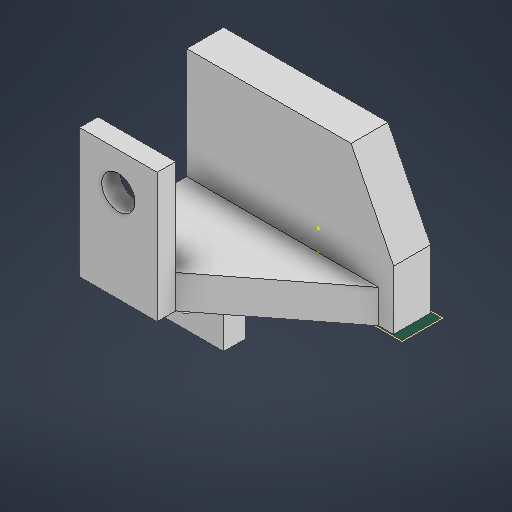
# Autodesk Inventor part: Part4
Saved by Autodesk Inventor 2026.2 (Build 302298000, 298)
## iProperties
Created: 2026-03-25
Part Number: Part4
Material: Generic
Document SubType Name: Modeling
Designer: LENOVO
Density: 1 g/cm^3
Appearance: Default
Author: LENOVO
Autodesk Inventor part; units mm, degrees
ref_plane "YZ Plane" through (0, 0, 0) normal (1, 0, 0) x (0, 1, 0)
ref_plane "XZ Plane" through (0, 0, 0) normal (0, 1, 0) x (-1, 0, 0)
ref_plane "XY Plane" through (0, 0, 0) normal (0, 0, 1) x (1, 0, 0)
sketch "Sketch1" plane through (0, 0, 0) normal (0, 0, 1) x (1, 0, 0)
  line L0 (40.6435, -29.4735) -> (-71.3565, -29.4735)
  line L1 (-71.3565, -29.4735) -> (-71.3565, 48.5265)
  line L2 (40.6435, -29.4735) -> (40.6435, 2.5265)
  line L3 (40.6435, 2.5265) -> (17.6435, 48.5265)
  line L4 (17.6435, 48.5265) -> (-71.3565, 48.5265)
  point P0 (0, 0)
  point P1 (40.6435, 100.5706)
  dimension "d0" = 112
  dimension "d1" = 78
  dimension "d5" = 32
  dimension "d8" = 23
  constraints: 10 end point, 4 coincident, 2 perpendicular, 1 horizontal, 1 vertical
  measures "d0" distance of L0.start L0.end
  measures "d1" distance of L0.end L1.end
  measures "d5" distance of L0.start L2.end
  measures "d8" distance from line of point (17.644, 48.527) L2
extrude "Extrusion1" add sketch "Sketch1" against normal blind 20
sketch "Sketch2" plane through (0, 0, 0) normal (0, 0, 1) x (1, 0, 0)
  point P0 (0, 0)
ref_plane "Work Plane1" through (-71.3565, -29.4735, 0) normal (0, -1, 0) x (1, 0, 0)
sketch "Sketch3" plane through (-71.3565, -29.4735, 0) normal (0, -1, 0) x (1, 0, 0)
  line L0 (0, 0) -> (0, 58)
  line L1 (0, 58) -> (42, 58)
  line L2 (42, 58) -> (42, 48)
  line L3 (42, 48) -> (104, 0)
  line L4 (112, 0) -> (89, 0) projected
  line L5 (0, 0) -> (104, 0)
  point P0 (71.3565, 0)
  dimension "d12" = 8
  dimension "d13" = 10
  dimension "d14" = 58
  dimension "d21" = 42
  constraints: 10 end point, 2 coincident, 2 perpendicular, 1 collinear, 1 point on line, 1 vertical
  measures "d12" distance of L4.start L3.end
  measures "d13" distance of L1.end L2.end
  measures "d14" distance of L0.start L0.end
  measures "d21" distance of L0.end L1.end
extrude "Extrusion2" add sketch "Sketch3" against normal blind 18
sketch "Sketch4" plane through (-71.3565, -29.4735, 0) normal (0, -1, 0) x (1, 0, 0)
  line L0 (0, 0) -> (0, 58) projected
  line L1 (0, 0) -> (32, 0)
  line L2 (32, 0) -> (32, 12)
  line L3 (32, 12) -> (0, 12)
  line L4 (0, 12) -> (0, 0)
  point P0 (71.3565, 0)
  point P1 (0, 12)
  dimension "d17" = 12
  dimension "d18" = 32
  constraints: 8 end point, 2 parallel, 1 horizontal, 1 perpendicular
  measures "d17" distance of L1.end L2.end
  measures "d18" distance of L2.end L3.end
extrude "Extrusion3" add sketch "Sketch4" along normal blind 42
sketch "Sketch5" plane through (-71.3565, -11.4735, 0) normal (0, 1, 0) x (1, 0, 0)
  point P0 (71.3565, 0)
sketch "Sketch6" plane through (-71.3565, -11.4735, 0) normal (0, 1, 0) x (1, 0, 0)
  line L0 (42, -48) -> (104, 0) projected
  line L1 (0, -58) -> (42, -58) projected
  line L2 (0, -58) -> (42, -58) projected
  line L3 (42, -58) -> (42, -48) projected
  line L4 (42, -48) -> (104, 0) projected
  line L5 (0, 0) -> (104, 0) projected
  line L6 (0, 0) -> (0, -58) projected
  line L7 (0, 0) -> (0, -58) projected
  line L8 (42, -58) -> (42, -48) projected
  line L9 (0, -58) -> (0, -12) projected
  line L10 (42, -58) -> (0, -58)
  line L11 (0, -58) -> (0, -48)
  line L12 (0, -48) -> (42, -48)
  line L13 (42, -48) -> (42, -58)
  point P0 (71.3565, 0)
  constraints: 8 end point, 2 parallel, 1 horizontal, 1 perpendicular, 1 point on line
extrude "Extrusion4" add sketch "Sketch6" along normal blind 52 contours L3 L1 L6 L12
sketch "Sketch7" plane through (-71.3565, -29.4735, 12) normal (0, 0, 1) x (1, 0, 0)
  line L0 (0, 0) -> (0, -42) projected
  circle A0 centre (10, -31) radius 4
  circle A1 centre (20, -19) radius 4
  point P0 (71.3565, 29.4735)
  point P1 (10, -42)
  point P2 (0, -31)
  point P3 (20, -42)
  point P4 (0, -19)
  dimension "d24" = 10
  dimension "d25" = 11
  dimension "d26" = 8
  dimension "d27" = 20
  dimension "d28" = 23
  dimension "d29" = 8
  constraints: 2 centre point, 2 coincident, 2 point on line
  measures "d24" distance of L0.end point (10, -42)
  measures "d25" distance of L0.end point (0, -31)
  measures "d26" diameter of A0
  measures "d27" distance of L0.end point (20, -42)
  measures "d28" distance of point (0, -19) L0.end
  measures "d29" diameter of A1
extrude "Extrusion5" cut sketch "Sketch7" against normal blind 52
sketch "Sketch8" plane through (-71.3565, -29.4735, 58) normal (0, 0, 1) x (1, 0, 0)
  line L0 (42, 0) -> (0, 0) projected
  line L1 (42, 0) -> (42, 70) projected
  line L2 (0, 70) -> (42, 70) projected
  line L3 (0, 0) -> (0, 70) projected
  line L4 (0, 70) -> (42, 70) projected
  circle A0 centre (21, 50) radius 9
  point P0 (71.3565, 29.4735)
  point P1 (0, 50)
  point P2 (21, 70)
  point P3 (21, 70)
  dimension "d32" = 21
  dimension "d33" = 20
  dimension "d34" = 18
  constraints: 2 coincident, 2 midpoint, 1 centre point, 1 point on line
  measures "d32" distance of L2.start point (21, 70)
  measures "d33" distance of L2.start point (0, 50)
  measures "d34" diameter of A0
extrude "Extrusion6" cut sketch "Sketch8" against normal blind 20 contours A0
body "Solid1"
